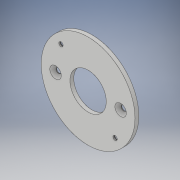
# Autodesk Inventor part: Lamp Centraaldoos Adapter v2
Saved by Autodesk Inventor 2019 (Build 230136000, 136)
## iProperties
Created: 2021-08-05
Part Number: Lamp Centraaldoos Adapter v2
Material: Generic
Document SubType Name: Modeling
Designer: Lix
Density: 1 g/cm^3
Appearance: Default
Author: Lix
Autodesk Inventor part; units mm, degrees
ref_plane "YZ Plane" through (0, 0, 0) normal (1, 0, 0) x (0, 1, 0)
ref_plane "XZ Plane" through (0, 0, 0) normal (0, 1, 0) x (-1, 0, 0)
ref_plane "XY Plane" through (0, 0, 0) normal (0, 0, 1) x (1, 0, 0)
sketch "Sketch1" plane through (0, 0, 0) normal (0, 0, 1) x (1, 0, 0)
  circle A0 centre (0, 0) radius 49
  dimension "d0" = 98
  constraints: 1 centre point, 1 coincident
  measures "d0" diameter of A0
extrude "Extrusion1" add sketch "Sketch1" along normal blind 4
sketch "Sketch2" plane through (0, 0, 4) normal (0, 0, 1) x (1, 0, 0)
  line L0 (-34, 0) -> (34, 0) construction
  line L1 (0, 27.5) -> (0, -27.5) construction
  point P0 (0, 0)
  point P1 (0, 0)
  dimension "d3" = 68
  dimension "d4" = 55
  constraints: 5 coincident, 4 end point, 2 midpoint, 1 horizontal, 1 vertical
  measures "d3" distance of L0.start L0.end
  measures "d4" distance of L1.start L1.end
hole "Hole1" at (-34, 0, 4) at (34, 0, 4) direction (0, 0, -1) diameter 5.5 depth 26.75 start extended yes countersink diameter 12 countersink angle 90
sketch "Sketch3" plane through (0, 0, 0) normal (0, 0, 1) x (1, 0, 0)
  line L0 (-35, 35) -> (35, 35) construction
  line L1 (35, 35) -> (35, -35) construction
  line L2 (35, -35) -> (-35, -35) construction
  line L3 (-35, -35) -> (-35, 35) construction
  line L4 (-35, 35) -> (35, -35) construction
  line L5 (35, 35) -> (-35, -35) construction
  circle A0 centre (0, 0) radius 60 construction
  line L6 (-28.2843, -28.2843) -> (28.2843, 28.2843) construction
  line L7 (0, 0) -> (24.0352, 0) construction
  point P0 (-28.2843, 28.2843)
  point P1 (28.2843, -28.2843)
  dimension "d12" = 70
  dimension "d13" = 70
  dimension "d14" = 120
  dimension "d15" = 80
  constraints: 16 end point, 4 midpoint, 3 coincident, 2 horizontal, 2 parallel, 2 symmetric about line, 1 centre point, 1 collinear, 1 perpendicular
  measures "d12" distance of L1.end L2.end
  measures "d13" distance of L0.end L1.end
  measures "d14" diameter of A0
  measures "d15" distance of L6.start L6.end
hole "Hole2" at (-28.2843, 28.2843, 0) at (28.2843, -28.2843, 0) direction (0, 0, 1) diameter 4.5 depth 26.75 start extended yes countersink diameter 10 countersink angle 90
sketch "Sketch4" plane through (0, 0, 4) normal (0, 0, 1) x (1, 0, 0)
  circle A0 centre (0, 0) radius 19
  dimension "d23" = 38
  constraints: 1 centre point, 1 coincident
  measures "d23" diameter of A0
extrude "Extrusion2" cut sketch "Sketch4" against normal blind 10
body "Solid1"
